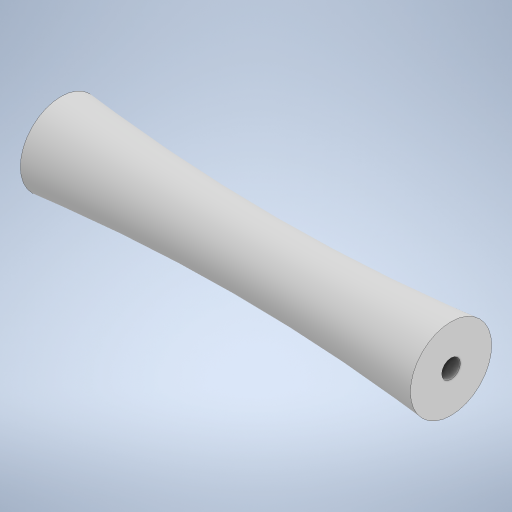
# Autodesk Inventor part: Roller
Saved by Autodesk Inventor 2024.2 (Build 282272000, 272)
## iProperties
Created: 2023-12-05
Part Number: Roller
Material: Generic
Document SubType Name: Modeling
Designer: felip
Density: 1 g/cm^3
Appearance: Default
Author: felip
Autodesk Inventor part; units mm, degrees
ref_plane "YZ Plane" through (0, 0, 0) normal (1, 0, 0) x (0, 1, 0)
ref_plane "XZ Plane" through (0, 0, 0) normal (0, 1, 0) x (-1, 0, 0)
ref_plane "XY Plane" through (0, 0, 0) normal (0, 0, 1) x (1, 0, 0)
sketch "Sketch1" plane through (0, 0, 0) normal (0, 1, 0) x (-1, 0, 0)
  line L0 (24, 18.5) -> (24, 23.5)
  line L1 (24, 23.5) -> (-24, 23.5)
  line L2 (-24, 23.5) -> (-24, 18.5)
  arc A0 (24, 18.5) -> (-24, 18.5) centre (0, -220.297) ccw
  point P0 (0, 0)
  dimension "d9" = 5
  dimension "d10" = 240
  constraints: 6 end point, 2 perpendicular, 2 point on circle, 1 centre point, 1 vertical
  measures "d9" distance of L0.start L0.end
  measures "d10" radius of A0
revolve "Revolution1" add sketch "Sketch1" angle 360 about axis through (-24, 0, 23.5) along (1, 0, 0)
sketch "Sketch2" plane through (24, 0, 23.5) normal (1, 0, 0) x (0, 0, -1)
  circle A0 centre (0, 0) radius 5 projected
  circle A1 centre (0, 0) radius 1.15
  point P0 (23.5, 0)
  dimension "d12" = 2.3
  constraints: 1 centre point, 1 coincident
  measures "d12" diameter of A1
extrude "Extrusion1" cut sketch "Sketch2" against normal blind 48 contours A1
body "Solid1"
